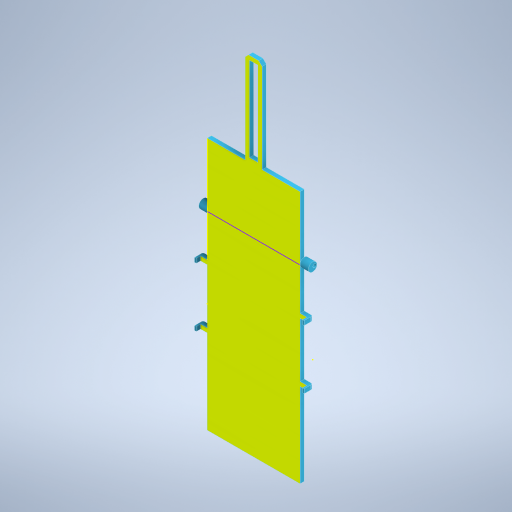
# Autodesk Inventor part: DSNDOOR 1
Saved by Autodesk Inventor 2024 (Build 280153000, 153)
## iProperties
Created: 2023-06-04
Part Number: DSNDOOR 1
Material: Titanium
Document SubType Name: Modeling
Designer: hithi
Density: 4.51 g/cm^3
Appearance: Turquoise
Author: hithi
Autodesk Inventor part; units mm, degrees
ref_plane "YZ Plane" through (0, 0, 0) normal (1, 0, 0) x (0, 1, 0)
ref_plane "XZ Plane" through (0, 0, 0) normal (0, 1, 0) x (-1, 0, 0)
ref_plane "XY Plane" through (0, 0, 0) normal (0, 0, 1) x (1, 0, 0)
sketch "Sketch1" plane through (0, 0, 0) normal (0, 0, 1) x (1, 0, 0)
  line L0 (0, 0) -> (110, 0)
  line L1 (110, 0) -> (110, 170)
  line L2 (110, 170) -> (0, 170)
  line L3 (0, 170) -> (0, 0)
  line L4 (45, 170) -> (65, 170)
  line L5 (65, 170) -> (65, 280)
  line L6 (65, 280) -> (45, 280)
  line L7 (45, 280) -> (45, 170)
  line L8 (50, 175) -> (60, 175)
  line L9 (60, 175) -> (60, 275)
  line L10 (60, 275) -> (50, 275)
  line L11 (50, 275) -> (50, 175)
  dimension "d0" = 110
  dimension "d1" = 170
  dimension "d2" = 20
  dimension "d3" = 110
  dimension "d4" = 10
  dimension "d5" = 100
  constraints: 24 end point, 6 parallel, 3 horizontal, 3 perpendicular, 1 point on line
  measures "d0" distance of L2.end L1.end
  measures "d1" distance of L1.end L0.end
  measures "d2" distance of L6.end L5.end
  measures "d3" distance of L5.end L4.end
  measures "d4" distance of L10.end L9.end
  measures "d5" distance of L9.end L8.end
extrude "Extrusion1" add sketch "Sketch1" along normal blind 5
chamfer "Chamfer1" distance 4 angle 45 2 edges at (45, 280, 2.5) (65, 280, 2.5)
sketch "Sketch2" plane through (110, 0, 0) normal (1, 0, 0) x (0, 0, -1)
  line L0 (0, 170) -> (0, 0) projected
  line L1 (0, 45) -> (-5, 45)
  line L2 (-5, 45) -> (-5, 40)
  line L3 (-5, 40) -> (0, 40)
  line L4 (0, 40) -> (0, 45)
  dimension "d11" = 5
  dimension "d12" = 5
  constraints: 8 end point, 2 parallel, 1 horizontal, 1 perpendicular, 1 point on line
  measures "d11" distance of L3.end L2.end
  measures "d12" distance of L2.end L1.end
sketch "Sketch3" plane through (0, 0, 0) normal (-1, 0, 0) x (0, 0, 1)
  line L0 (5, 0) -> (5, 170) projected
  line L1 (0, 170) -> (0, 0) projected
  line L2 (5, 39.9453) -> (0, 39.9453)
  line L3 (0, 39.9453) -> (0, 44.9453)
  line L4 (0, 44.9453) -> (5, 44.9453)
  line L5 (5, 44.9453) -> (5, 39.9453)
  dimension "d13" = 5
  constraints: 8 end point, 2 parallel, 2 point on line, 1 horizontal, 1 perpendicular
  measures "d13" distance of L2.end L3.end
extrude "Extrusion2" add sketch "Sketch3" along normal blind 10
extrude "Extrusion3" add sketch "Sketch2" along normal blind 10
sketch "Sketch4" plane through (0, 0, 5) normal (0, 0, 1) x (1, 0, 0)
  line L0 (0, 44.9453) -> (-10, 44.9453) projected
  line L1 (0, 39.9453) -> (-10, 39.9453) projected
  line L2 (-10, 44.9453) -> (-8, 44.9453)
  line L3 (-8, 44.9453) -> (-8, 39.9453)
  line L4 (-8, 39.9453) -> (-10, 39.9453)
  line L5 (-10, 39.9453) -> (-10, 44.9453)
  line L6 (120, 45) -> (120, 40) projected
  line L7 (120, 45) -> (118, 45)
  line L8 (118, 45) -> (118, 39.9453)
  line L9 (118, 39.9453) -> (120, 39.9453)
  line L10 (120, 39.9453) -> (120, 45)
  point P0 (0, 0)
  dimension "d18" = 2
  dimension "d19" = 2
  constraints: 16 end point, 4 parallel, 2 horizontal, 2 perpendicular, 2 point on line
  measures "d18" distance of L3.end L4.end
  measures "d19" distance of L9.end L8.end
extrude "Extrusion4" add sketch "Sketch4" along normal blind 5 contours L3 L1 L5 L0
sketch "Sketch5" plane through (0, 0, 5) normal (0, 0, 1) x (1, 0, 0)
  line L0 (120, 45) -> (120, 40) projected
  line L1 (110, 45) -> (120, 45) projected
  line L2 (120, 40) -> (118, 40)
  line L3 (118, 40) -> (118, 45)
  line L4 (118, 45) -> (120, 45)
  line L5 (120, 45) -> (120, 40)
  point P0 (0, 0)
  dimension "d22" = 2
  constraints: 8 end point, 2 parallel, 1 horizontal, 1 perpendicular, 1 point on line
  measures "d22" distance of L3.end L4.end
extrude "Extrusion5" add sketch "Sketch5" along normal blind 5
fillet "Fillet1" radius 2 2 edges at (120, 42.5, 0) (-10, 42.4453, 0)
sketch "Sketch6" plane through (0, 0, 0) normal (0, -1, 0) x (1, 0, 0)
  line L0 (110, 0) -> (110, 5) projected
  line L1 (0, 0) -> (110, 0)
  line L2 (110, 0) -> (110, 5)
  line L3 (110, 5) -> (0, 5)
  line L4 (0, 5) -> (0, 0)
  constraints: 8 end point, 2 parallel, 1 horizontal, 1 perpendicular
extrude "Extrusion6" add sketch "Sketch6" along normal blind 90
sketch "Sketch7" plane through (0, 0, 5) normal (0, 0, 1) x (1, 0, 0)
  line L0 (0, 170) -> (0, 44.9453) projected
  line L1 (0, 94.7501) -> (109.4357, 94.7501)
  point P0 (0, 0)
  constraints: 2 end point, 1 horizontal, 1 point on line
sketch "Sketch8" plane through (110, 40, 5) normal (1, 0, 0) x (0, 0, -1)
  line L0 (5, 0) -> (5, -130) projected
  line L1 (5, -65) -> (0, -65)
  line L2 (0, -65) -> (0, -70)
  line L3 (0, -70) -> (5, -70)
  line L4 (5, -70) -> (5, -65)
  point P0 (5, -40)
  dimension "d28" = 5
  dimension "d29" = 5
  constraints: 8 end point, 2 parallel, 1 horizontal, 1 midpoint, 1 perpendicular
  measures "d28" distance of L3.end L2.end
  measures "d29" distance of L2.end L1.end
sketch "Sketch9" plane through (0, 39.9453, 0) normal (-1, 0, 0) x (0, 0, 1)
  line L0 (5, 0.0547) -> (5, -129.9453) projected
  line L1 (5, -65) -> (0, -65)
  line L2 (0, -65) -> (0, -70)
  line L3 (0, -70) -> (5, -70)
  line L4 (5, -70) -> (5, -65)
  point P0 (0, -39.9453)
  dimension "d30" = 5
  dimension "d31" = 5
  constraints: 8 end point, 2 parallel, 1 horizontal, 1 perpendicular, 1 point on line
  measures "d30" distance of L3.end L2.end
  measures "d31" distance of L2.end L1.end
extrude "Extrusion7" add sketch "Sketch9" along normal blind 10
extrude "Extrusion8" add sketch "Sketch8" along normal blind 10
sketch "Sketch10" plane through (0, 0, 5) normal (0, 0, 1) x (1, 0, 0)
  line L0 (0, -25.0547) -> (-10, -25.0547) projected
  line L1 (0, -30.0547) -> (-10, -30.0547) projected
  line L2 (-10, -25.0547) -> (-8, -25.0547)
  line L3 (-8, -25.0547) -> (-8, -30.0547)
  line L4 (-8, -30.0547) -> (-10, -30.0547)
  line L5 (-10, -30.0547) -> (-10, -25.0547)
  line L6 (120, -25) -> (120, -30) projected
  line L7 (120, -25) -> (118, -25)
  line L8 (118, -25) -> (118, -30)
  line L9 (118, -30) -> (120, -30)
  line L10 (120, -30) -> (120, -25)
  point P0 (0, 0)
  dimension "d36" = 2
  dimension "d37" = 2
  constraints: 16 end point, 4 parallel, 2 horizontal, 2 perpendicular, 1 point on line
  measures "d36" distance of L3.end L4.end
  measures "d37" distance of L9.end L8.end
extrude "Extrusion9" add sketch "Sketch10" along normal blind 5
fillet "Fillet2" radius 2 2 edges at (120, -27.5, 0) (-10, -27.5547, 0)
sketch "Sketch11" plane through (110, 170, 5) normal (1, 0, 0) x (0, 0, -1)
  line L0 (5, -125) -> (5, 0) projected
  circle A0 centre (5, -74.823) radius 5.0652
  circle A1 centre (7.3498, -74.823) radius 2.0605
  point P0 (5, -170)
  constraints: 2 centre point, 1 point on line
extrude "Extrusion10" add sketch "Sketch11" along normal blind 10
sketch "Sketch12" plane through (120, 95.177, 0) normal (1, 0, 0) x (0, 0, -1)
  point P0 (0, -95.177)
sketch "Sketch13" plane through (110, 170, 5) normal (-1, 0, 0) x (0, 0, 1)
  circle A0 centre (-7.3498, -74.823) radius 2.0605 projected
  circle A1 centre (-7.3498, -74.823) radius 2.0605
  point P0 (-5, -170)
  constraints: 1 centre point, 1 coincident
extrude "Extrusion11" add sketch "Sketch13" along normal blind 110
sketch "Sketch14" plane through (0, 95.177, -2.3498) normal (-1, 0, 0) x (0, 0, 1)
  circle A0 centre (0, 0) radius 2.0605
  circle A1 centre (0, 0) radius 2.0605 projected
  circle A2 centre (2.0605, 0) radius 5.309
  point P0 (2.3498, -95.177)
  constraints: 2 centre point, 1 horizontal alignment, 1 other
extrude "Extrusion12" add sketch "Sketch14" along normal blind 10
sketch "Sketch15" plane through (0, 170, 0) normal (-1, 0, 0) x (0, 0, 1)
  line L0 (0, 0) -> (0, -69.5219) projected
  line L1 (5, 0) -> (5, -74.3661) projected
  circle A0 centre (-2.3126, -29.4971) radius 1.6501
  point P0 (0, -170)
  constraints: 1 centre point
sketch "Sketch16" plane through (0, -90, 0) normal (0, -1, 0) x (1, 0, 0)
  line L0 (0, 0) -> (-8, 0) projected
  line L1 (0, 0) -> (110, 0)
  line L2 (110, 0) -> (110, 5)
  line L3 (110, 5) -> (0, 5)
  line L4 (0, 5) -> (0, 0)
  constraints: 8 end point, 2 parallel, 1 horizontal, 1 perpendicular
extrude "Extrusion13" add sketch "Sketch16" along normal blind 40
body "Solid1"
